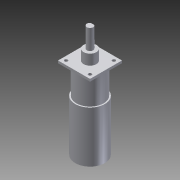
# Autodesk Inventor part: mr85vel 3 etapas
Saved by Autodesk Inventor 2011 (Build 150239000, 239)
## iProperties
Created: 2010-04-19
Part Number: mr85vel 3 etapas
Document SubType Name: Modeling
Designer: lucio
Density: 0.94 g/cm^3
Material: UHMW, White
Mass: 102.512 g
Surface Area: 165.171 cm^2
Volume: 109.055 cm^3
Author: lucio
Autodesk Inventor part; units mm, degrees
ref_plane "YZ Plane" through (0, 0, 0) normal (1, 0, 0) x (0, 1, 0)
ref_plane "XZ Plane" through (0, 0, 0) normal (0, 1, 0) x (-1, 0, 0)
ref_plane "XY Plane" through (0, 0, 0) normal (0, 0, 1) x (1, 0, 0)
sketch "Sketch1" plane through (0, 0, 0) normal (0, 0, 1) x (1, 0, 0)
  line L0 (0, 0) -> (40, 0)
  line L1 (40, 0) -> (40, 40)
  line L2 (40, 40) -> (0, 40)
  line L3 (0, 40) -> (0, 0)
  dimension "d0" = 40
  dimension "d1" = 40
  constraints: 8 end point, 2 parallel, 1 horizontal, 1 perpendicular
  measures "d0" distance of L2.end L1.end
  measures "d1" distance of L1.end L0.end
extrude "Extrusion1" add sketch "Sketch1" along normal blind 3
sketch "Sketch2" plane through (0, 0, 3) normal (0, 0, 1) x (1, 0, 0)
  line L0 (40, 0) -> (0, 0) projected
  line L1 (40, 40) -> (40, 0) projected
  line L2 (35, 5) -> (5, 5)
  line L3 (5, 5) -> (5, 35)
  line L4 (5, 35) -> (35, 35)
  line L5 (35, 35) -> (35, 5)
  circle A0 centre (20, 20) radius 8
  dimension "d4" = 30
  dimension "d5" = 30
  dimension "d6" = 5
  dimension "d7" = 5
  dimension "d8" = 16
  constraints: 8 end point, 2 parallel, 1 centre point, 1 horizontal, 1 perpendicular
  measures "d4" distance of L3.end L4.end
  measures "d5" distance of L2.end L3.end
  measures "d6" distance between parallel lines of L0 L2
  measures "d7" distance between parallel lines of L1 L5
  measures "d8" diameter of A0
extrude "Extrusion2" add sketch "Sketch2" along normal blind 13 contours A0
sketch "Sketch3" plane through (0, 0, 3) normal (0, 0, 1) x (1, 0, 0)
  line L0 (40, 0) -> (0, 0) projected
  line L1 (40, 40) -> (40, 0) projected
  line L2 (5, 5) -> (35, 5)
  line L3 (35, 5) -> (35, 35)
  line L4 (35, 35) -> (5, 35)
  line L5 (5, 35) -> (5, 5)
  dimension "d11" = 30
  dimension "d12" = 30
  dimension "d13" = 5
  dimension "d14" = 5
  constraints: 8 end point, 2 parallel, 1 horizontal, 1 perpendicular
  measures "d11" distance of L4.end L3.end
  measures "d12" distance of L3.end L2.end
  measures "d13" distance between parallel lines of L0 L2
  measures "d14" distance between parallel lines of L1 L3
hole "Hole1" at (5, 5, 3) at (35, 5, 3) at (35, 35, 3) at (5, 35, 3) direction (0, 0, -1) diameter 4 end through all
sketch "Sketch4" plane through (20, 20, 16) normal (0, 0, 1) x (1, 0, 0)
  circle A0 centre (0, 0) radius 8 projected
  circle A1 centre (0, 0) radius 4
  point P0 (-20, -20)
  dimension "d22" = 8
  constraints: 1 centre point, 1 coincident
  measures "d22" diameter of A1
extrude "Extrusion3" add sketch "Sketch4" along normal blind 25 contours A1
sketch "Sketch5" plane through (20, 20, 41) normal (0, 0, 1) x (1, 0, 0)
  circle A0 centre (0, 0) radius 4 projected
  line L0 (-4, 0) -> (4, 0)
  line L1 (4, 0) -> (4, 4)
  line L2 (4, 4) -> (-4, 4)
  line L3 (-4, 4) -> (-4, 0)
  line L4 (-4, 4) -> (4, 4)
  line L5 (4, 4) -> (4, 3.2)
  line L6 (4, 3.2) -> (-4, 3.2)
  line L7 (-4, 3.2) -> (-4, 4)
  point P0 (-20, -20)
  dimension "d25" = 0.8
  constraints: 16 end point, 4 parallel, 2 horizontal, 2 perpendicular, 1 horizontal alignment, 1 point on line, 1 other
  measures "d25" distance of L4.end L5.end
extrude "Extrusion4" cut sketch "Sketch5" against normal blind 21 contours L6 L3 L2 A0 | A0 L6 | A0 L2 L1 L6
sketch "Sketch6" plane through (0, 0, 0) normal (0, 0, -1) x (-1, 0, 0)
  circle A0 centre (-20, 20) radius 17
  dimension "d28" = 34
  constraints: 1 centre point
  measures "d28" diameter of A0
extrude "Extrusion5" add sketch "Sketch6" along normal blind 35
sketch "Sketch7" plane through (20, 20, -35) normal (0, 0, -1) x (-1, 0, 0)
  circle A0 centre (0, 0) radius 17 projected
  circle A1 centre (0, 0) radius 18.5
  point P0 (20, -20)
  dimension "d31" = 37
  constraints: 1 centre point, 1 coincident
  measures "d31" diameter of A1
extrude "Extrusion6" add sketch "Sketch7" along normal blind 64 contours A0 | A1
body "Solid1"
